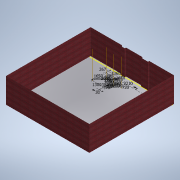
# Autodesk Inventor part: Entorno
Saved by Autodesk Inventor 2020 (Build 240168000, 168)
## iProperties
Created: 2019-10-05
Part Number: Entorno
Material: Genérico
Document SubType Name: Modeling
Designer: dasa1
Density: 1 g/cm^3
Appearance: Textura gruesa - Blanco
Author: dasa1
Autodesk Inventor part; units mm, degrees
ref_plane "YZ Plane" through (0, 0, 0) normal (1, 0, 0) x (0, 1, 0)
ref_plane "XZ Plane" through (0, 0, 0) normal (0, 1, 0) x (-1, 0, 0)
ref_plane "XY Plane" through (0, 0, 0) normal (0, 0, 1) x (1, 0, 0)
sketch "Boceto1" plane through (0, 0, 0) normal (0, 1, 0) x (-1, 0, 0)
  line L0 (0, 0) -> (0, -650) construction
  line L1 (0, -650) -> (4000, -650) construction
  line L2 (4000, -650) -> (-6000, -650)
  line L3 (-6000, -650) -> (-6000, 9350)
  line L4 (-6000, 9350) -> (4000, 9350)
  line L5 (4000, 9350) -> (4000, -650)
  dimension "d1" = 650
  dimension "d2" = 4000
  dimension "d3" = 10000
  dimension "d4" = 10000
  constraints: 12 end point, 2 parallel, 2 perpendicular, 1 horizontal, 1 vertical
  measures "d1" distance of L0.start L0.end
  measures "d2" distance of L0.end L1.end
  measures "d3" distance of L3.end L4.end
  measures "d4" distance of L2.end L3.end
extrude "Extrusión1" add sketch "Boceto1" along normal blind 1
sketch "Boceto3" plane through (0, 1, 0) normal (0, 1, 0) x (1, 0, 0)
  line L0 (-4000, 650) -> (-4000, -9350) construction
  line L1 (-4000, -9350) -> (6000, -9350) construction
  line L2 (6000, -9350) -> (6000, 650) construction
  line L3 (6000, 650) -> (-4000, 650) construction
  line L4 (6000, 650) -> (6000, 651)
  line L5 (-4000, 650) -> (-4000, -9350) projected
  line L6 (-4001, 650) -> (-4001, -9350)
  line L7 (-4001, -9350) -> (-4000, -9350)
  line L8 (-4000, -9350) -> (-4000, 650)
  line L9 (-4000, -9350) -> (6000, -9350)
  line L10 (6000, -9350) -> (6000, -9351)
  line L11 (6000, -9351) -> (-4000, -9351)
  line L12 (-4000, -9351) -> (-4000, -9350)
  line L13 (6000, -9350) -> (6001, -9350)
  line L14 (6001, -9350) -> (6001, 650)
  line L15 (6001, 650) -> (6000, 650) construction
  line L16 (6000, 650) -> (6000, -9350)
  line L17 (-50, 651) -> (200, 651)
  line L18 (200, 651) -> (-200, 651)
  line L19 (0, 651) -> (250, 651) construction
  line L20 (250, 651) -> (-249, 651) construction
  line L21 (-250, 651) -> (-249, 651) construction
  line L22 (-249, 651) -> (-249, 801)
  line L23 (-249, 801) -> (-250, 801)
  line L24 (-250, 800) -> (-250, 651)
  line L25 (250, 651) -> (249, 651) construction
  line L26 (249, 651) -> (249, 801)
  line L27 (249, 801) -> (250, 801)
  line L28 (250, 800) -> (250, 651)
  line L29 (249, 651) -> (-249, 651)
  line L30 (6000, 801) -> (6000, 800) construction
  line L31 (249, 800) -> (249, 801)
  line L32 (6001, 650) -> (6000, 650) construction
  line L33 (6000, 650) -> (6000, 800)
  line L34 (6000, 800) -> (6001, 800) construction
  line L35 (6001, 800) -> (6001, 650)
  line L36 (-250, 801) -> (-4000, 801)
  line L37 (-4000, 801) -> (-4000, 800) construction
  line L38 (-4000, 800) -> (-250, 800)
  line L39 (-250, 800) -> (-250, 801) construction
  line L40 (-4000, 801) -> (-4001, 801)
  line L41 (-4001, 801) -> (-4001, 650)
  line L42 (-4000, 651) -> (-4000, 800)
  line L43 (-250, 651) -> (-250, 650)
  line L44 (250, 651) -> (250, 650)
  line L45 (6000, 650) -> (-4000, 650) projected
  line L46 (6000, 801) -> (6001, 801)
  line L47 (6001, 801) -> (6001, 800)
  line L48 (6001, 800) -> (6000, 800) construction
  line L49 (6000, 800) -> (6000, 801) construction
  line L50 (2210, 650) -> (2210, 200) construction
  line L51 (2210, 200) -> (3040, 200) construction
  line L52 (3040, 200) -> (3040, 650) construction
  line L53 (3040, 650) -> (2210, 650) construction
  line L54 (2210, 650) -> (2211, 650)
  line L55 (2211, 651) -> (2211, 800)
  line L56 (2211, 800) -> (2210, 800) construction
  line L57 (2210, 800) -> (2210, 650)
  line L58 (3040, 650) -> (3039, 650)
  line L59 (3039, 651) -> (3039, 800)
  line L60 (3039, 800) -> (3040, 800) construction
  line L61 (3040, 800) -> (3040, 650)
  line L62 (2211, 650) -> (3039, 650)
  line L63 (3039, 650) -> (3039, 651) construction
  line L64 (3039, 651) -> (2211, 651)
  line L65 (2211, 651) -> (2211, 650) construction
  line L66 (2210, 800) -> (250, 800)
  line L67 (6000, 800) -> (3040, 800)
  line L68 (2211, 801) -> (2211, 800)
  line L69 (3039, 800) -> (3039, 801)
  line L70 (249, 801) -> (2211, 801)
  line L71 (3039, 801) -> (6000, 801)
  line L72 (-4000, 651) -> (-4000, 650)
  point P0 (0, 0)
  point P1 (-4000, -9350)
  point P2 (-4000, -9350)
  point P3 (-2000, -9350)
  point P4 (6000, 650)
  point P5 (6000, 650)
  dimension "d7" = 1
  dimension "d8" = 1
  dimension "d9" = 1
  dimension "d10" = 1
  dimension "d24" = 10000
  dimension "d32" = 0
  dimension "d34" = 0
  dimension "d36" = 10000
  dimension "d37" = 8000
  dimension "d38" = 10000
  dimension "d39" = 8000
  dimension "d40" = 10000
  dimension "d41" = 8000
  dimension "d42" = 0
  dimension "d81" = 250
  dimension "d82" = 500
  dimension "d83" = 1
  dimension "d84" = 150
  dimension "d85" = 1
  dimension "d86" = 150
  dimension "d87" = 1
  dimension "d88" = 1
  dimension "d89" = 90
  dimension "d90" = 90
  dimension "d94" = 0
  dimension "d95" = 0
  dimension "d96" = 151
  dimension "d97" = 5751
  dimension "d98" = 4250
  dimension "d99" = 0
  dimension "d100" = 1
  dimension "d101" = 0
  dimension "d102" = 0
  dimension "d103" = 150
  dimension "d104" = 5800
  dimension "d105" = 6050
  dimension "d106" = 0
  dimension "d107" = 1
  dimension "d108" = 0
  dimension "d111" = 1
  dimension "d112" = 1
  dimension "d113" = 1
  dimension "d114" = 90
  dimension "d115" = 151
  dimension "d116" = 150
  dimension "d117" = 2961
  constraints: 134 end point, 28 parallel, 16 perpendicular, 13 horizontal, 4 point on line, 1 collinear, 1 midpoint, 2 other
  measures "d7" distance of L4.end L4.start
  measures "d8" distance of L7.end L6.end
  measures "d9" distance of L9.end L10.end
  measures "d10" distance of L15.end L14.end
  measures "d24" distance between parallel lines of L3 L7
  measures "d32" distance from line of point (6000, 650) L3
  measures "d34" distance from line of point (6000, 650) L3
  measures "d36" distance from line of point (-4000, -9350) L3
  measures "d38" distance from line of point (-4000, -9350) L3
  measures "d40" distance from line of point (-2000, -9350) L3
  measures "d41" distance from line of point (-2000, -9350) L2
  measures "d42" distance between parallel lines of L2 L16
  measures "d81" distance of L19.start L19.end
  measures "d82" distance of L19.end L21.start
  measures "d83" distance of L23.end L22.end
  measures "d84" distance of L20.end L22.end
  measures "d85" distance of L26.end L27.end
  measures "d86" distance of L25.end L26.end
  measures "d87" distance of L30.start L30.end
  measures "d88" distance of L37.end L36.end
  measures "d89" angle to the sketch x axis of L44
  measures "d90" angle to the sketch x axis of L8
  measures "d94" vertical extent of L32
  measures "d95" distance between parallel lines of L2 L30
  measures "d96" distance between parallel lines of L3 L27
  measures "d97" distance between parallel lines of L2 L26
  measures "d98" distance between parallel lines of L0 L28
  measures "d99" distance between parallel lines of L0 L42
  measures "d100" distance from line of L4.end L3
  measures "d101" distance from line of point (6000, 650) L2
  measures "d102" distance from line of point (6000, 650) L2
  measures "d103" distance from line of L31.start L3
  measures "d104" distance from line of L17.end L2
  measures "d105" distance from line of L17.start L2
  measures "d106" distance from line of L43.end L3
  measures "d107" distance from line of L42.start L3
  measures "d108" distance from line of L6.start L3
  measures "d111" distance of L56.end L55.end
  measures "d112" distance of L59.end L60.end
  measures "d113" distance of L59.start L62.end
  measures "d114" angle of L53 L4
  measures "d115" distance between parallel lines of L53 L46
  measures "d116" distance between parallel lines of L53 L66
  measures "d117" distance from line of L58.end L2
extrude "Extrusión2" add sketch "Boceto3" along normal blind 3000 contours L4 L33 L67 L61 L45 L57 L66 L28 L44 L43 L24 L38 L42 L72 L5 L7 L6 L41 L40 L36 L23 L22 L29 L18 L17 L26 L27 L70 L68 L55 L64 L59 L69 L71 L46 L47 L35 L14 L13 L16 | L10 L11 L12 L9
sketch "Boceto4" plane through (0, 1, 0) normal (0, 1, 0) x (1, 0, 0)
  line L0 (0, 0) -> (370, 0) construction
  line L1 (0, 0) -> (2210, 0) construction
  line L2 (0, 0) -> (-385, 0) construction
  line L3 (0, 185) -> (0, 0) construction
  line L4 (0, 0) -> (-1260, 0) construction
  line L5 (0, 360) -> (0, 0) construction
  line L6 (0, 0) -> (250, 0) construction
  line L7 (250, 0) -> (250, -820) construction
  line L8 (250, -820) -> (0, -820) construction
  line L9 (0, -820) -> (0, 0) construction
  line L10 (0, 0) -> (-300, 0) construction
  line L11 (-300, 0) -> (-300, -1247) construction
  line L12 (-300, -1247) -> (0, -1247) construction
  line L13 (0, -1247) -> (0, 0) construction
  line L14 (0, 0) -> (30, 0) construction
  line L15 (30, 0) -> (30, -2220) construction
  line L16 (30, -2220) -> (0, -2220) construction
  line L17 (0, -2220) -> (0, 0) construction
  line L18 (0, 0) -> (1200, 0) construction
  line L19 (1200, 0) -> (1200, -720) construction
  line L20 (1200, -720) -> (0, -720) construction
  line L21 (0, -720) -> (0, 0) construction
  line L22 (0, 0) -> (-650, 0) construction
  line L23 (-650, 0) -> (-650, -650) construction
  line L24 (-650, -650) -> (0, -650) construction
  line L25 (0, -650) -> (0, 0) construction
  line L26 (6000, 650) -> (-4000, 650) projected
  line L27 (0, 0) -> (-1300, 0) construction
  line L28 (-1300, 0) -> (-1300, -1650) construction
  line L29 (-1300, -1650) -> (0, -1650) construction
  line L30 (0, -1650) -> (0, 0) construction
  line L31 (0, 0) -> (515, 0) construction
  line L32 (515, 0) -> (515, -1475) construction
  line L33 (515, -1475) -> (0, -1475) construction
  line L34 (0, -1475) -> (0, 0) construction
  line L35 (0, 0) -> (485, 0) construction
  line L36 (485, 0) -> (485, -1240) construction
  line L37 (485, -1240) -> (0, -1240) construction
  line L38 (0, -1240) -> (0, 0) construction
  line L39 (0, 0) -> (495, 0) construction
  line L40 (495, 0) -> (495, -972) construction
  line L41 (495, -972) -> (0, -972) construction
  line L42 (0, -972) -> (0, 0) construction
  line L43 (0, 0) -> (-385, 0) construction
  line L44 (-385, 0) -> (-385, -185) construction
  line L45 (-385, -185) -> (0, -185) construction
  line L46 (0, -185) -> (0, 0) construction
  line L47 (0, 0) -> (-1360, 0) construction
  line L48 (-1360, 0) -> (-1360, 267) construction
  line L49 (-1360, 267) -> (0, 267) construction
  line L50 (0, 267) -> (0, 0) construction
  line L51 (30, 0) -> (3030, 0) construction
  line L52 (0, 0) -> (-1414.2136, -1414.2136)
  line L53 (0, 0) -> (2000, 0) construction
  line L54 (0, 0) -> (30, -33.541)
  line L55 (30, -33.541) -> (-33.6396, 30.0986)
  line L56 (-33.6396, 30.0986) -> (-1447.8532, -1384.115)
  line L57 (-385, -185) -> (-1360, 0) construction
  point P0 (0, 650)
  dimension "d13" = 370
  dimension "d14" = 2210
  dimension "d19" = 250
  dimension "d20" = 820
  dimension "d21" = 300
  dimension "d22" = 1247
  dimension "d47" = 30
  dimension "d48" = 2220
  dimension "d49" = 1200
  dimension "d50" = 720
  dimension "d51" = 650
  dimension "d52" = 650
  dimension "d54" = 650
  dimension "d56" = 1300
  dimension "d57" = 1650
  dimension "d58" = 515
  dimension "d59" = 1475
  dimension "d60" = 485
  dimension "d61" = 1240
  dimension "d62" = 495
  dimension "d63" = 972
  dimension "d64" = 385
  dimension "d65" = 185
  dimension "d66" = 1360
  dimension "d67" = 267
  dimension "d70" = 2000
  dimension "d71" = 135
  dimension "d72" = 45
  dimension "d73" = 90
  dimension "d74" = 2000
  constraints: 82 end point, 30 horizontal, 22 parallel, 13 perpendicular, 13 vertical, 2 point on line, 1 coincident, 1 horizontal alignment, 6 other
  measures "d19" distance of L7.end L8.end
  measures "d20" distance of L6.end L7.end
  measures "d21" distance of L12.end L11.end
  measures "d22" distance of L11.end L10.end
  measures "d47" distance of L15.end L16.end
  measures "d48" distance of L14.end L15.end
  measures "d49" distance of L19.end L20.end
  measures "d50" distance of L18.end L19.end
  measures "d51" distance of L24.end L23.end
  measures "d52" distance of L23.end L22.end
  measures "d56" distance of L29.end L28.end
  measures "d57" distance of L28.end L27.end
  measures "d58" distance of L32.end L33.end
  measures "d59" distance of L31.end L32.end
  measures "d60" distance of L36.end L37.end
  measures "d61" distance of L35.end L36.end
  measures "d62" distance of L40.end L41.end
  measures "d63" distance of L39.end L40.end
  measures "d64" distance of L45.end L44.end
  measures "d65" distance of L44.end L43.end
  measures "d66" distance of L48.end L49.end
  measures "d67" distance of L47.end L48.end
  measures "d71" angle of L52 L53
  measures "d73" distance of L54.end L55.end
  measures "d74" distance of L55.end L56.end
sketch "Boceto5" plane through (0, 0, 0) normal (0, -1, 0) x (1, 0, 0)
  line L0 (-249, -801) -> (-4001, -801) projected
  line L1 (-249, -651) -> (-249, -801) projected
  line L2 (250, -650) -> (250, -800) projected
  line L3 (250, -800) -> (2210, -800) projected
  line L4 (2210, -800) -> (2210, -650) projected
  line L5 (6001, -801) -> (3039, -801) projected
  line L6 (3039, -801) -> (3039, -651) projected
  line L7 (6000, -800) -> (6000, -650) projected
  line L8 (-4000, -650) -> (-4000, -800) projected
  line L9 (6000, -650) -> (-4000, -650) projected
  line L10 (6001, -801) -> (3039, -801) projected
  line L11 (6000, -650) -> (3040, -650) projected
  line L12 (6001, -801) -> (3040, -801)
  line L13 (3040, -801) -> (3040, -650)
  line L14 (3040, -650) -> (6001, -650)
  line L15 (6001, -650) -> (6001, -801)
  line L16 (250, -800) -> (2210, -800) projected
  line L17 (249, -801) -> (249, -651) projected
  line L18 (2210, -800) -> (249, -800)
  line L19 (249, -800) -> (249, -651)
  line L20 (249, -651) -> (2210, -651)
  line L21 (2210, -651) -> (2210, -800)
  line L22 (-250, -650) -> (-4000, -650) projected
  line L23 (-249, -801) -> (-4000, -801)
  line L24 (-4000, -801) -> (-4000, -650)
  line L25 (-4000, -650) -> (-249, -650)
  line L26 (-249, -650) -> (-249, -801)
  point P0 (0, 0)
  point P1 (-249, -650)
  constraints: 24 end point, 6 parallel, 3 horizontal, 3 perpendicular
extrude "Extrusión3" add sketch "Boceto5" against normal blind 1 contours L0 L24 L8 L9 L26 L1 | L20 L4 L3 L2 | L2 L18 L17 L20 | L5 L13 L9 L14 L15
